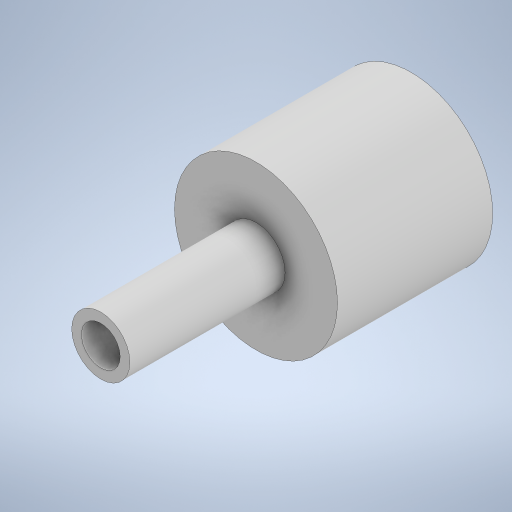
# Autodesk Inventor part: roller_inner
Saved by Autodesk Inventor 2023 (Build 270158000, 158)
## iProperties
Created: 2022-07-07
Part Number: roller_inner
Material: Generic
Document SubType Name: Modeling
Designer: Zayed
Density: 1 g/cm^3
Appearance: Default
Author: Zayed
## iProperties of the stored document roller_inner_3DPrint.ipt
Created: 2022-07-07
Part Number: roller_inner_3DPrint
Material: Generic
Document SubType Name: Modeling
Designer: Zayed
Density: 1 g/cm^3
Appearance: Default
Author: Zayed
Autodesk Inventor part; units mm, degrees
ref_plane "YZ Plane" through (0, 0, 0) normal (1, 0, 0) x (0, 1, 0)
ref_plane "XZ Plane" through (0, 0, 0) normal (0, 1, 0) x (-1, 0, 0)
ref_plane "XY Plane" through (0, 0, 0) normal (0, 0, 1) x (1, 0, 0)
sketch "Sketch1" plane through (0, 0, 0) normal (0, 0, 1) x (1, 0, 0)
  circle A0 centre (0, 0) radius 10.5
  circle A1 centre (0, 0) radius 2.5
  circle A2 centre (0, 0) radius 3.75
  dimension "d0" = 21
  dimension "d1" = 5
  dimension "d4" = 7.5
  constraints: 3 centre point, 3 coincident
  measures "d0" diameter of A0
  measures "d1" diameter of A1
  measures "d4" diameter of A2
extrude "Extrusion6" add sketch "Sketch1" along normal blind 20 contours A2
extrude "Extrusion7" add sketch "Sketch1" against normal blind 20 contours A0 | A2
body "Solid4"
